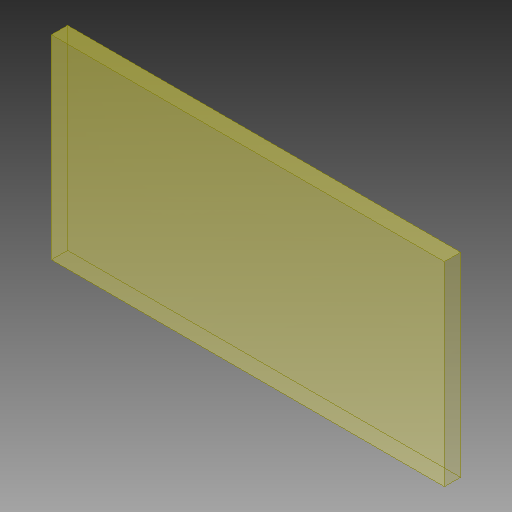
# Autodesk Inventor part: surround_front back
Saved by Autodesk Inventor 2018.1 (Build 221171000, 171)
## iProperties
Created: 2017-07-30
Part Number: surround_front back
Material: PVC-Piping
Document SubType Name: Modeling
Designer: Tom
Density: 1.4 g/cm^3
Appearance: Clear - Yellow
Mass: 39.312 g
Surface Area: 154.56 cm^2
Volume: 28.08 cm^3
Author: Tom
Autodesk Inventor part; units mm, degrees
ref_plane "YZ Plane" through (0, 0, 0) normal (1, 0, 0) x (0, 1, 0)
ref_plane "XZ Plane" through (0, 0, 0) normal (0, 1, 0) x (-1, 0, 0)
ref_plane "XY Plane" through (0, 0, 0) normal (0, 0, 1) x (1, 0, 0)
sketch "Sketch1" plane through (0, 0, 0) normal (0, 0, 1) x (1, 0, 0)
  line L0 (0, 0) -> (121, 0)
  line L1 (121, 0) -> (121, 60)
  line L2 (121, 60) -> (0, 60)
  line L3 (0, 60) -> (0, 0)
  dimension "d0" = 121
  dimension "d1" = 60
  constraints: 8 end point, 2 parallel, 1 horizontal, 1 perpendicular
  measures "d0" distance of L2.end L1.end
  measures "d1" distance of L1.end L0.end
extrude "Extrusion1" add sketch "Sketch1" along normal blind 5
equation "\"d0\" = tankw + 2 * slack + 2 * surroundt + 2 * pvct"
equation "\"d1\" = surroundh"
equation "\"d2\" = surroundt"
equation "\"lcsd\" = 19.05"
equation "\"lcwd1\" = 25"
equation "\"lcwd2\" = 34"
equation "\"lch1\" = 39"
equation "\"lcwd3\" = 43"
equation "\"dia1\" = 6"
equation "\"td\" = 18"
equation "\"bhh\" = 6"
equation "\"sw\" = 25"
equation "\"sh\" = 31"
equation "\"spacert\" = 2"
equation "\"pvct\" = 5"
equation "\"tankl\" = 379"
equation "\"dia4\" = 11"
equation "\"dia3\" = 8"
equation "\"play\" = 9"
equation "\"holeh\" = 26"
equation "\"surroundh\" = 60"
equation "\"slack\" = 0.5"
equation "\"surroundt\" = 5"
equation "\"play2\" = 3"
equation "\"diaoverflow\" = 25"
equation "\"diaair\" = 32"
equation "\"diaph\" = 32"
equation "\"diacucl\" = 32"
equation "\"diawater\" = 25"
equation "\"diasurroundhole\" = 42"
equation "\"diagrate\" = 12"
equation "\"gratespacing\" = 12.02082"
equation "\"bottomdist\" = 9.6355"
equation "\"sidedist\" = 13.9375"
equation "\"diahcl\" = 32"
equation "\"bracketwtop\" = 6"
equation "\"bracketwbottom\" = 6"
equation "\"nett\" = 1"
equation "\"nethole\" = 16"
equation "\"netside\" = 3.5"
equation "\"nettop\" = 7"
equation "\"netholespacing\" = 2"
equation "\"diaetape\" = 32"
equation "\"tankw\" = 100"
body "Solid1"
